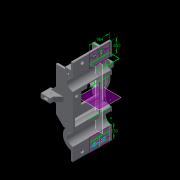
# Autodesk Inventor part: Extruder Holder V2
Saved by Autodesk Inventor 2014 (Build 180170000, 170)
## iProperties
Created: 2015-07-07
Part Number: Extruder Holder V2
Material: Generic
Document SubType Name: Modeling
Designer: Scott
Density: 1 g/cm^3
Appearance: Default
Author: Scott
Autodesk Inventor part; units mm, degrees
ref_plane "YZ Plane" through (0, 0, 0) normal (1, 0, 0) x (0, 1, 0)
ref_plane "XZ Plane" through (0, 0, 0) normal (0, 1, 0) x (-1, 0, 0)
ref_plane "XY Plane" through (0, 0, 0) normal (0, 0, 1) x (1, 0, 0)
ref_plane "Work Plane1" through (0, -60, 0) normal (0, 0, 1) x (-1, 0, 0)
sketch "Sketch1" plane through (0, -60, 0) normal (0, 0, 1) x (-1, 0, 0)
  circle A0 centre (0, 0) radius 4 projected
  circle A1 centre (0, -60) radius 4 projected
  circle A2 centre (0, -60) radius 7.5
  circle A3 centre (0, 0) radius 7.5
  circle A4 centre (0, -60) radius 12.7
  circle A5 centre (0, 0) radius 12.7
  dimension "d0" = 15
  dimension "d1" = 15
  dimension "d2" = 25.4
  dimension "d3" = 25.4
  constraints: 4 centre point, 4 coincident
  measures "d0" diameter of A2
  measures "d1" diameter of A3
  measures "d2" diameter of A4
  measures "d3" diameter of A5
extrude "Extrusion1" add sketch "Sketch1" along normal mid plane 25 contours A4 | A5
sketch "Sketch2" plane through (0, 0, 12.5) normal (0, 0, 1) x (1, 0, 0)
  circle A0 centre (0, 0) radius 12.7 projected
  circle A1 centre (0, -60) radius 7.5 projected
  circle A2 centre (0, -60) radius 12.7 projected
  circle A3 centre (0, 0) radius 7.5 projected
  circle A4 centre (0, 0) radius 12.7 projected
  line L0 (0, -72.7) -> (12.7, -72.7)
  line L1 (12.7, -72.7) -> (12.7, 12.706)
  line L2 (12.7, 12.706) -> (0, 12.7)
  circle A5 centre (0, -60) radius 12.7 projected
  arc A6 (0, -72.7) -> (12.7, -60) centre (0, -60) ccw
  arc A7 (12.7, 0) -> (0, 12.7) centre (0, 0) ccw
  constraints: 6 end point, 6 point on circle, 2 centre point, 2 horizontal, 2 point on line, 2 vertical alignment, 1 horizontal alignment, 1 perpendicular, 3 other
extrude "Extrusion2" add sketch "Sketch2" against normal blind 25 contours A0 L2 L1 | L1 L0 A2
sketch "Sketch3" plane through (12.7, 12.706, 12.5) normal (-0.0004741, 0.9999999, 0) x (0.9999999, 0.0004741, 0)
  line L0 (0, 0) -> (-12.7, 0) projected
  line L1 (0, 0) -> (0, 25) projected
  line L2 (-12.7, 25) -> (0, 25) projected
  line L3 (-12.7, 0) -> (-12.7, 25) projected
  point P0 (-12.706, 12.5)
sketch "Sketch4" plane through (0, -60, -12.5) normal (0, 0, -1) x (-1, 0, 0)
  line L0 (-12.7, 72.706) -> (-12.7, 60) projected
  line L1 (0, 72.7) -> (0, -16.7444)
  line L2 (0, -16.7444) -> (-14.0452, -16.7444)
  line L3 (-14.0452, -16.7444) -> (-14.0452, 76.9468)
  line L4 (-14.0452, 76.9468) -> (0, 72.7)
  constraints: 8 end point, 2 parallel, 1 perpendicular
extrude "Extrusion3" cut sketch "Sketch4" against normal blind 52.3875
sketch "Sketch5" plane through (0, 7.5, -12.5) normal (1, 0, 0) x (0, 0, -1)
  line L0 (-25, 0) -> (-25, 5.2) projected
  line L1 (0, 0) -> (-25, 0) projected
  line L2 (0, 5.2) -> (0, 0) projected
  line L3 (-25, 5.2) -> (0, 5.2) projected
  line L4 (-25, 0) -> (-0.0064, 0)
  line L5 (-0.0064, 0) -> (-0.0064, 16.51)
  line L6 (-0.0064, 16.51) -> (-25, 16.51)
  line L7 (-25, 16.51) -> (-25, 0)
  line L8 (-12.5, 5.2) -> (-12.5032, 16.51)
  line L9 (-12.5016, 10.855) -> (-25, 10.855)
  circle A0 centre (-18.7508, 10.855) radius 2.2225
  line L10 (-0.0064, 10.855) -> (-12.5016, 10.855)
  circle A1 centre (-6.254, 10.855) radius 2.2225
  line L11 (0, -20.2) -> (-25, -20.2) projected
  line L12 (-25, -54.8) -> (0, -54.8) projected
  line L13 (-12.5, -20.2) -> (-12.5, -54.8)
  line L14 (-12.5, -37.5) -> (-25, -37.5)
  line L15 (-25, -75) -> (0, -75) projected
  line L16 (-25, -80.2) -> (-25, -75) projected
  line L17 (-25, -80.2) -> (0, -80.2) projected
  line L18 (0, -75) -> (0, -80.2) projected
  line L19 (-25, -75) -> (0, -75)
  line L20 (0, -75) -> (0, -91.51)
  line L21 (0, -91.51) -> (-25, -91.51)
  line L22 (-25, -91.51) -> (-25, -75)
  line L23 (-12.5, -80.2) -> (-12.5, -91.51)
  line L24 (-25, -85.855) -> (-12.5, -85.855)
  line L25 (-12.5, -85.855) -> (0, -85.855)
  circle A2 centre (-18.75, -85.855) radius 2.2225
  circle A3 centre (-6.25, -85.855) radius 2.2225
  point P0 (-12.5, -7.5)
  dimension "d10" = 24.9936
  dimension "d11" = 16.51
  dimension "d12" = 4.445
  dimension "d13" = 4.445
  dimension "d14" = 16.51
  dimension "d15" = 4.445
  dimension "d16" = 4.445
  constraints: 32 end point, 13 midpoint, 5 perpendicular, 4 centre point, 4 parallel, 4 point on line, 2 horizontal, 1 collinear
  measures "d10" distance of L6.end L5.end
  measures "d11" distance of L5.end L4.end
  measures "d12" diameter of A0
  measures "d13" diameter of A1
  measures "d14" distance of L19.end L20.end
  measures "d15" diameter of A2
  measures "d16" diameter of A3
extrude "Extrusion4" add sketch "Sketch5" against normal blind 2.54
ref_plane "Work Plane2" through (0, -30, -12.5) normal (0, -1, 0) x (1, 0, 0)
sketch "Sketch6" plane through (0, -30, -12.5) normal (0, -1, 0) x (1, 0, 0)
  line L0 (0, 0) -> (0, 25) projected
  line L1 (0, 25) -> (0, 25) projected
  line L2 (0, 25) -> (0, 0) projected
  line L3 (0, 0) -> (0, 0) projected
  line L4 (-7.5, 25) -> (0, 25) projected
  line L5 (0, 0) -> (0, 25) projected
  line L6 (0, 25) -> (0, 25) projected
  line L7 (0, 25) -> (0, 0) projected
  line L8 (0, 0) -> (0, 0) projected
  line L9 (-2.54, 0) -> (-2.54, 25) projected
  line L10 (0, 25) -> (-2.54, 25) projected
  line L11 (0, 25) -> (0, 0) projected
  line L12 (-2.54, 0) -> (0, 0) projected
  line L13 (-7.5, 0) -> (-7.5, 25) projected
  line L14 (-7.5, 0) -> (-10.04, 0)
  line L15 (-10.04, 0) -> (-10.04, 43)
  line L16 (-7.5, 43) -> (-7.5, 0)
  line L17 (-10.04, 0) -> (-21.54, 0)
  line L18 (-21.54, 0) -> (-21.54, -2.54)
  line L19 (-21.54, -2.54) -> (-7.5, -2.54)
  line L20 (-7.5, -2.54) -> (-7.5, 0)
  line L21 (-10.04, 43) -> (-21.54, 43)
  line L22 (-21.54, 43) -> (-21.54, 45.54)
  line L23 (-21.54, 45.54) -> (-7.5, 45.54)
  line L24 (-7.5, 45.54) -> (-7.5, 43)
  point P0 (0, 12.5)
  dimension "d21" = 2.54
  dimension "d22" = 43
  dimension "d23" = 11.5
  dimension "d24" = 2.54
  dimension "d25" = 11.5
  dimension "d26" = 2.54
  constraints: 22 end point, 7 perpendicular, 3 parallel, 1 collinear
  measures "d21" distance of L13.start L14.end
  measures "d22" distance of L14.end L15.end
  measures "d23" distance of L14.end L17.end
  measures "d24" distance of L17.end L18.end
  measures "d25" distance of L15.end L21.end
  measures "d26" distance of L21.end L22.end
extrude "Extrusion6" add sketch "Sketch6" along normal blind 21.59 and the other way blind 42.2275 contours L14 L15 L21 L22 L23 L24 L16 L13 | L20 L19 L18 L17 L14
sketch "Sketch7" plane through (0, -51.59, -12.5) normal (0, -1, 0) x (1, 0, 0)
  line L0 (-10.04, 43) -> (-21.54, 43)
  line L1 (-21.54, 43) -> (-21.54, 0)
  line L2 (-21.54, 0) -> (-10.04, 0)
  line L3 (-10.04, 0) -> (-10.04, 43)
  point P0 (0, 12.5)
  constraints: 8 end point, 2 parallel, 1 horizontal, 1 perpendicular
extrude "Extrusion7" cut sketch "Sketch7" along normal mid plane 152.4
sketch "Sketch8" plane through (0, -60, 12.5) normal (0, 0, 1) x (1, 0, 0)
  line L0 (-7.5, 8.41) -> (-9.5164, 8.41) projected
  arc A0 (-9.5164, 8.41) -> (-2.54, -12.4434) centre (0, 0) ccw projected
  line L1 (-2.54, -24.01) -> (-2.54, -12.4434) projected
  line L2 (0, -24.01) -> (-2.54, -24.01) projected
  line L3 (0, -24.01) -> (0, -7.5) projected
  arc A1 (0, 7.5) -> (0, -7.5) centre (0, 0) ccw projected
  line L4 (0, 7.5) -> (0, 12.7) projected
  arc A2 (0, 12.7) -> (-7.5, 10.2489) centre (0, 0) ccw projected
  line L5 (-7.5, 10.2489) -> (-7.5, 8.41) projected
  line L6 (-7.5, 70.2489) -> (-7.5, 60) projected
  arc A3 (0, 67.5) -> (-7.5, 60) centre (0, 60) ccw projected
  line L7 (0, 84.01) -> (0, 67.5) projected
  line L8 (0, 84.01) -> (-2.54, 84.01) projected
  line L9 (-2.54, 72.4434) -> (-2.54, 84.01) projected
  arc A4 (-2.54, 72.4434) -> (-7.5, 70.2489) centre (0, 60) ccw projected
  line L10 (-7.5, 60) -> (-7.5, 49.7511) projected
  arc A5 (-7.5, 49.7511) -> (0, 47.3) centre (0, 60) ccw projected
  line L11 (0, 47.3) -> (0, 52.5) projected
  arc A6 (-7.5, 60) -> (0, 52.5) centre (0, 60) ccw projected
extrude "Extrusion8" add sketch "Sketch8" along normal up to surface (20.54 mm away)
sketch "Sketch9" plane through (0, -60, -12.5) normal (0, 0, -1) x (-1, 0, 0)
  line L0 (9.5164, 8.41) -> (7.5, 8.41) projected
  line L1 (7.5, 8.41) -> (7.5, 10.2489) projected
  arc A0 (7.5, 10.2489) -> (0, 12.7) centre (0, 0) ccw projected
  line L2 (0, 12.7) -> (0, 7.5) projected
  arc A1 (0, -7.5) -> (0, 7.5) centre (0, 0) ccw projected
  line L3 (0, -24.01) -> (0, -7.5) projected
  line L4 (0, -24.01) -> (2.54, -24.01) projected
  line L5 (2.54, -12.4434) -> (2.54, -24.01) projected
  arc A2 (2.54, -12.4434) -> (9.5164, 8.41) centre (0, 0) ccw projected
  arc A3 (8.3332, 63.0967) -> (2.2038, 68.6125) centre (0, 60) ccw projected
  line L6 (7.5, 60) -> (7.5, 70.2489) projected
  arc A4 (7.5, 70.2489) -> (2.54, 72.4434) centre (0, 60) ccw projected
  line L7 (2.54, 72.7) -> (2.54, 72.4434) projected
  line L8 (0, 72.7) -> (2.54, 72.7) projected
  line L9 (0, 72.7) -> (0, 67.5) projected
  arc A5 (7.5, 60) -> (0, 67.5) centre (0, 60) ccw projected
  line L10 (2.54, 72.7) -> (0, 72.7) projected
  line L11 (2.54, 84.01) -> (2.54, 72.7) projected
  line L12 (0, 84.01) -> (2.54, 84.01) projected
  line L13 (0, 72.7) -> (0, 84.01) projected
  line L14 (7.5, 49.7511) -> (7.5, 60) projected
  arc A6 (0, 52.5) -> (7.5, 60) centre (0, 60) ccw projected
  line L15 (0, 52.5) -> (0, 47.3) projected
  arc A7 (0, 47.3) -> (7.5, 49.7511) centre (0, 60) ccw projected
extrude "Extrusion9" add sketch "Sketch9" along normal up to surface (2.54 mm away)
sketch "Sketch10" plane through (-10.04, -51.59, -12.5) normal (-1, 0, 0) x (0, 0, 1)
  line L0 (43, 0) -> (33.221, 0)
  line L1 (33.221, 0) -> (33.221, 29.845)
  line L2 (33.221, 29.845) -> (43, 29.845)
  line L3 (43, 29.845) -> (43, 0)
  circle A0 centre (33.221, 29.845) radius 1.905
  line L4 (31.316, 29.845) -> (27.506, 29.845)
  line L5 (27.506, 29.845) -> (27.506, 42.545)
  line L6 (27.506, 42.545) -> (27.506, 17.145)
  line L7 (27.506, 17.145) -> (3.376, 17.145)
  line L8 (3.376, 17.145) -> (3.376, 42.545)
  line L9 (3.376, 42.545) -> (27.506, 42.545)
  point P0 (12.5, 51.59)
  dimension "d39" = 3.81
  dimension "d37" = 9.779
  dimension "d38" = 29.845
  dimension "d40" = 3.81
  dimension "d41" = 12.7
  dimension "d42" = 25.4
  dimension "d43" = 24.13
  constraints: 20 end point, 4 parallel, 4 perpendicular, 1 coincident, 1 collinear, 1 horizontal, 1 horizontal alignment, 2 other
  measures "d37" distance of L1.end L2.end
  measures "d38" distance of L0.end L1.end
  measures "d40" distance of L4.start L4.end
  measures "d41" distance of L4.end L5.end
  measures "d42" distance of L5.end L6.end
  measures "d43" distance of L6.end L7.end
extrude "Extrusion10" cut sketch "Sketch10" against normal blind 75.565 contours A0 L2 L1 | L1 L2 A0 | L6 L7 L8 L9 L5
sketch "Sketch11" plane through (-7.5, 12.2275, -15.04) normal (0, 0, -1) x (-1, 0, 0)
  arc A0 (-4.96, -84.6709) -> (2.0164, -63.8175) centre (-7.5, -72.2275) ccw projected
  line L0 (14.04, -63.8175) -> (2.0164, -63.8175) projected
  line L1 (-7.5, -24.9275) -> (-7.5, -21.2725) projected
  arc A1 (-7.5, -24.9275) -> (0, -22.4764) centre (-7.5, -12.2275) ccw projected
  line L2 (0, -46.6725) -> (0, -22.4764) projected
  line L3 (2.54, -46.6725) -> (0, -46.6725) projected
  line L4 (2.54, -21.2725) -> (2.54, -46.6725) projected
  line L5 (2.54, -21.2725) -> (-7.5, -21.2725) projected
  line L6 (2.54, 0) -> (2.54, -63.8175) projected
  line L7 (14.04, -63.8175) -> (2.54, -63.8175) projected
  line L8 (14.04, 0) -> (14.04, -63.8175) projected
  line L9 (2.54, 0) -> (14.04, 0) projected
  line L10 (2.54, -63.8175) -> (2.54, -64.4501)
  line L11 (2.54, -63.8175) -> (2.0164, -63.8175)
  line L12 (2.0164, -63.8175) -> (2.54, -64.4501)
  constraints: 6 end point, 1 collinear, 1 perpendicular, 1 point on circle
extrude "Extrusion11" add sketch "Sketch11" against normal up to surface (48.08 mm away) contours A0 L0 L10
fillet "Fillet1" radius 6.35 2 edges at (-7.5, -49.7511, -13.77) (-7.5, -49.7511, 10.27)
fillet "Fillet2" radius 6.35 2 edges at (-7.5, 10.2489, 10.27) (-7.5, 10.2489, -13.77)
chamfer "Chamfer1" distance 9.525 angle 45 2 edges at (-21.54, -51.59, -13.77) (-21.54, -51.59, 31.77)
sketch "Sketch14" plane through (0, -60, 33.04) normal (0, 0, 1) x (1, 0, 0)
  line L0 (-7.5, 49.7511) -> (-7.5, 19.0153) projected
  line L1 (-21.54, 72.2275) -> (-21.54, 17.935) projected
  line L2 (-10.04, 36.35) -> (-10.04, 40.16) projected
  line L3 (-10.04, 38.255) -> (-7.5, 38.255)
  line L4 (-7.5, 38.255) -> (-11.0275, 38.255)
  line L5 (-11.0275, 38.255) -> (-21.1875, 38.255)
  line L6 (-21.54, 38.255) -> (-27.382, 38.255)
  line L7 (-27.382, 36.985) -> (-21.54, 36.985)
  line L8 (-21.54, 36.985) -> (-21.54, 39.525)
  line L9 (-21.54, 39.525) -> (-27.382, 39.525)
  line L10 (-27.382, 39.525) -> (-27.382, 36.985)
  line L11 (-27.382, 36.985) -> (-21.54, 39.525) construction
  line L12 (-21.54, 36.985) -> (-27.382, 39.525) construction
  line L13 (-30.3665, 35.3975) -> (-18.5555, 35.3975)
  line L14 (-18.5555, 35.3975) -> (-18.5555, 41.1125)
  line L15 (-18.5555, 41.1125) -> (-30.3665, 41.1125)
  line L16 (-30.3665, 41.1125) -> (-30.3665, 35.3975)
  line L17 (-30.3665, 35.3975) -> (-18.5555, 41.1125) construction
  line L18 (-18.5555, 35.3975) -> (-30.3665, 41.1125) construction
  point P0 (-24.461, 38.255)
  dimension "d61" = 10.16
  dimension "d62" = 5.842
  dimension "d63" = 5.842
  dimension "d64" = 2.54
  dimension "d65" = 11.811
  dimension "d66" = 5.715
  constraints: 32 end point, 6 midpoint, 4 parallel, 3 collinear, 3 perpendicular, 2 horizontal, 2 point on line
  measures "d61" distance of L4.end L5.end
  measures "d62" distance of L6.start L6.end
  measures "d63" distance of L9.end L8.end
  measures "d64" distance of L8.end L7.end
  measures "d65" distance of L15.end L14.end
  measures "d66" distance of L14.end L13.end
extrude "Extrusion14" add sketch "Sketch14" along normal blind 10.16 contours L1 L15 L14 L13 | L9 L10 L7 L1 L13 L16 L15
sketch "Sketch15" plane through (0, -60, 33.04) normal (0, 0, -1) x (-1, 0, 0)
  line L0 (30.3665, 41.1125) -> (21.54, 41.1125)
  line L1 (21.54, 41.1125) -> (21.54, 35.3975)
  line L2 (21.54, 35.3975) -> (30.3665, 35.3975)
  line L3 (30.3665, 35.3975) -> (30.3665, 41.1125)
  point P0 (0, 60)
  constraints: 8 end point, 2 parallel, 1 horizontal, 1 perpendicular
extrude "Extrusion15" add sketch "Sketch15" along normal up to surface (2.54 mm away)
chamfer "Chamfer2" distance 6.35 angle 45 1 edges at (-18.5555, -21.745, 33.04)
chamfer "Chamfer3" distance 6.35 angle 45 2 edges at (-21.54, -24.6025, 31.77) (-21.54, -18.8875, 31.77)
sketch "Sketch16" plane through (0, 0, -15.04) normal (0, 0, -1) x (-1, 0, 0)
  line L0 (21.54, -42.065) -> (12.015, -51.59) projected
  line L1 (21.54, 12.2275) -> (21.54, -42.065) projected
  line L2 (7.5, 12.2275) -> (21.54, 12.2275) projected
  arc A0 (3.6503, 12.1641) -> (7.5, 12.2275) centre (5.4755, 18.2461) ccw projected
  arc A1 (3.6503, 12.1641) -> (2.54, 12.4434) centre (0, 0) ccw projected
  line L3 (2.54, 24.01) -> (2.54, 12.4434) projected
  line L4 (0, 24.01) -> (2.54, 24.01) projected
  line L5 (0, 7.5) -> (0, 24.01) projected
  arc A2 (0, -7.5) -> (0, 7.5) centre (0, 0) ccw projected
  line L6 (0, -12.7) -> (0, -7.5) projected
  arc A3 (0, -12.7) -> (7.5, -10.2489) centre (0, 0) ccw projected
  line L7 (7.5, -10.2489) -> (7.5, -40.9847) projected
  arc A4 (0.7667, -47.3232) -> (7.5, -40.9847) centre (1.15, -40.9847) ccw projected
  arc A5 (0.7667, -47.3232) -> (0, -47.3) centre (0, -60) ccw projected
  line L8 (0, -52.5) -> (0, -47.3) projected
  arc A6 (0, -67.5) -> (0, -52.5) centre (0, -60) ccw projected
  line L9 (0, -84.01) -> (0, -67.5) projected
  line L10 (2.54, -84.01) -> (0, -84.01) projected
  line L11 (2.54, -72.4434) -> (2.54, -84.01) projected
  arc A7 (2.54, -72.4434) -> (10.04, -52.2226) centre (0, -60) ccw projected
  line L12 (10.04, -52.2226) -> (10.04, -51.59) projected
  line L13 (12.015, -51.59) -> (10.04, -51.59) projected
  line L14 (11, -18.441) -> (11, -2.5) projected
sketch "Sketch17" plane through (-21.54, 12.2275, -15.04) normal (-1, 0, 0) x (0, 0, 1)
  line L0 (2.54, 0) -> (2.54, -54.2925) projected
  line L1 (0, 0) -> (0, -54.2925) projected
  line L2 (5.916, -21.2725) -> (30.046, -21.2725) projected
  line L3 (30.046, -46.6725) -> (5.916, -46.6725) projected
  line L4 (0, -21.2725) -> (-7.62, -21.2725)
  line L5 (-7.62, -21.2725) -> (-7.62, -46.6725)
  line L6 (-7.62, -46.6725) -> (0, -46.6725)
  line L7 (0, -46.6725) -> (0, -21.2725)
  line L8 (0, -21.2725) -> (0, -17.4625)
  line L9 (0, -17.4625) -> (-11.43, -17.4625)
  line L10 (-11.43, -17.4625) -> (-11.43, -46.6725)
  line L11 (-11.43, -46.6725) -> (-11.43, -50.4825)
  line L12 (-11.43, -50.4825) -> (0, -50.4825)
  line L13 (0, -21.8952) -> (2.54, -21.8952)
  line L14 (0, -17.4625) -> (2.54, -17.4625)
  line L15 (2.54, -21.8952) -> (2.54, -17.4625)
  line L16 (0, -50.4825) -> (2.54, -50.4825)
  line L17 (0, -46.6725) -> (2.54, -46.6725)
  line L18 (2.54, -46.6725) -> (2.54, -50.4825)
  line L19 (0, -21.2725) -> (2.54, -21.2725)
  point P0 (15.04, -12.2275)
  dimension "d77" = 7.62
  dimension "d78" = 25.4
  dimension "d79" = 3.81
  dimension "d80" = 11.43
  dimension "d81" = 3.81
  constraints: 32 end point, 9 point on line, 8 perpendicular, 4 parallel, 2 collinear, 1 horizontal
  measures "d77" distance of L6.end L5.end
  measures "d78" distance of L5.end L4.end
  measures "d79" distance of L4.start L8.end
  measures "d80" distance of L8.end L9.end
  measures "d81" distance of L10.end L11.end
extrude "Extrusion16" add sketch "Sketch17" along normal mid plane 18.0975 contours L0 L19 L1 L14 | L1 L4 L5 L6 L12 L11 L10 L9 | L0 L16 L1 L17
sketch "Sketch18" plane through (-30.5888, -9.045, -22.66) normal (0, 0, 1) x (1, 0, 0)
  line L0 (3.2068, -13.97) -> (3.2068, -11.43) projected
  line L1 (3.2068, -11.43) -> (9.0488, -11.43) projected
  line L2 (9.0488, -11.43) -> (9.0488, -13.97) projected
  line L3 (9.0488, -13.97) -> (3.2068, -13.97) projected
  line L4 (0.2223, -15.5575) -> (12.0332, -15.5575) projected
  line L5 (12.0332, -15.5575) -> (12.0332, -9.8425) projected
  line L6 (12.0332, -9.8425) -> (0.2223, -9.8425) projected
  line L7 (0.2223, -9.8425) -> (0.2223, -15.5575) projected
  point P0 (30.5888, 9.045)
extrude "Extrusion17" add sketch "Sketch18" against normal blind 13.97
sketch "Sketch19" plane through (-21.54, -34.445, -12.5) normal (-1, 0, 0) x (0, 0, 1)
  line L0 (-2.54, 0) -> (0, 0) projected
  line L1 (0, 25.4) -> (0, 0) projected
  line L2 (0, 25.4) -> (-2.54, 25.4) projected
  line L3 (-2.54, 25.4) -> (-2.54, 0) projected
  line L4 (-2.54, 21.745) -> (3.376, 21.745) projected
  line L5 (-2.54, 0) -> (0, 0) projected
  line L6 (0, 25.4) -> (0, 0) projected
  line L7 (0, 25.4) -> (-2.54, 25.4) projected
  line L8 (-2.54, 25.4) -> (-2.54, 0) projected
  point P0 (12.5, 34.445)
extrude "Extrusion18" cut sketch "Sketch19" against normal blind 6.0325
fillet "Fillet3" radius 7.9375 8 edges at (-17.0156, -34.445, -22.66) (-26.0644, -34.445, -22.66) (-17.0156, -38.255, -26.47) (-26.0644, -38.255, -26.47) (-17.0156, -5.235, -26.47) (-26.0644, -5.235, -26.47) (-17.0156, -9.045, -22.66) (-26.0644, -9.045, -22.66)
chamfer "Chamfer5" distance 4.7625 angle 45 2 edges at (-12.4912, -7.1432, -15.04) (-12.4912, -36.3468, -15.04)
chamfer "Chamfer6" distance 7.9375 angle 45 1 edges at (-21.54, -5.235, -13.77)
chamfer "Chamfer7" distance 4.7625 angle 45 1 edges at (-18.5555, -21.745, -26.47)
chamfer "Chamfer8" distance 6.35 angle 45 2 edges at (-30.5888, -36.35, -12.5) (-30.5888, -7.14, -12.5)
sketch "Sketch20" plane through (0, -60, 33.04) normal (0, 0, 1) x (1, 0, 0)
  arc A0 (-7.5, 19.0153) -> (-0.7667, 12.6768) centre (-1.15, 19.0153) ccw projected
  line L0 (-5.0623, 14.0136) -> (-8.4175, 14.0136)
  line L1 (-8.4175, 14.0136) -> (-8.4175, 19.653)
  line L2 (-8.4175, 19.653) -> (-5.0623, 19.653)
  line L3 (-5.0623, 19.653) -> (-5.0623, 14.0136)
  constraints: 8 end point, 2 parallel, 1 horizontal, 1 perpendicular, 1 point on circle
extrude "Extrusion19" cut sketch "Sketch20" against normal blind 56.8325
sketch "Sketch21" plane through (-10.04, 12.2275, 30.5) normal (0, 0, -1) x (-1, 0, 0)
  line L0 (21.1166, -48.5775) -> (21.1166, -35.8775) projected
  line L1 (0.96, -35.8775) -> (21.1166, -35.8775) projected
  line L2 (0.96, -48.5775) -> (21.1166, -48.5775) projected
  line L3 (21.1166, -48.5775) -> (11.5, -48.5775)
  line L4 (11.5, -48.5775) -> (11.5, -54.2925)
  line L5 (11.5, -54.2925) -> (21.1166, -54.2925)
  line L6 (21.1166, -54.2925) -> (21.1166, -48.5775)
  point P0 (-10.04, -12.2275)
  constraints: 8 end point, 2 parallel, 1 horizontal, 1 perpendicular
extrude "Extrusion20" cut sketch "Sketch21" along normal blind 56.8325
fillet "Fillet4" radius 1.5875 1 edges at (-21.54, -36.35, -18.0956)
sketch "Sketch22" plane through (-30.3665, -24.6025, -36.63) normal (0, -1, 0) x (1, 0, 0)
  circle A0 centre (5.9055, 5.08) radius 0.635
  line L0 (2.4765, 69.67) -> (2.4765, 67.13) projected
  line L1 (2.4765, 69.67) -> (18.161, 69.67) projected
  line L2 (11.811, 76.02) -> (18.161, 69.67) projected
  line L3 (11.811, 76.02) -> (11.811, 79.83) projected
  line L4 (0, 79.83) -> (11.811, 79.83) projected
  line L5 (0, 79.83) -> (0, 67.13) projected
  line L6 (0, 67.13) -> (2.4765, 67.13) projected
  circle A1 centre (6.5405, 73.48) radius 0.635
  point P0 (30.3665, 36.63)
  dimension "d109" = 1.27
  dimension "d110" = 1.27
  constraints: 2 centre point
  measures "d109" diameter of A0
  measures "d110" diameter of A1
extrude "Extrusion21" cut sketch "Sketch22" against normal blind 56.8325 contours A0 | A1
sketch "Sketch23" plane through (-2.54, 7.5, -12.5) normal (-1, 0, 0) x (0, 0, 1)
  line L0 (-2.54, -79.9434) -> (45.54, -79.9434) projected
  line L1 (-2.54, -79.9434) -> (-2.54, -91.51) projected
  line L2 (45.54, -91.51) -> (-2.54, -91.51) projected
  line L3 (45.54, -91.51) -> (45.54, -79.9434) projected
  line L4 (45.54, 4.9434) -> (-2.54, 4.9434) projected
  line L5 (45.54, 4.9434) -> (45.54, 16.51) projected
  line L6 (0.0064, 16.51) -> (45.54, 16.51) projected
  line L7 (0.0064, 16.51) -> (0.0064, 5.2) projected
  line L8 (0.0064, 5.2) -> (0, 5.2) projected
  line L9 (0, 5.2) -> (0, 16.51) projected
  line L10 (0, 16.51) -> (-2.54, 16.51) projected
  line L11 (-2.54, 16.51) -> (-2.54, 4.9434) projected
  line L12 (21.5, -79.9434) -> (21.5, -91.51)
  line L13 (21.5, -85.7267) -> (45.54, -85.7267)
  line L14 (21.5, -85.7267) -> (-2.54, -85.7267)
  circle A0 centre (9.48, -85.7267) radius 2.2225
  circle A1 centre (33.52, -85.7267) radius 2.2225
  line L15 (21.5, 16.51) -> (21.5, 4.9434)
  line L16 (21.5, 10.7267) -> (-2.54, 10.7267)
  line L17 (21.5, 10.7267) -> (45.54, 10.7267)
  circle A2 centre (9.48, 10.7267) radius 2.2225
  circle A3 centre (33.52, 10.7267) radius 2.2225
  point P0 (12.5, -7.5)
  dimension "d113" = 4.445
  dimension "d114" = 4.445
  dimension "d115" = 4.445
  dimension "d116" = 4.445
  constraints: 13 midpoint, 12 end point, 4 centre point, 1 point on line
  measures "d113" diameter of A0
  measures "d114" diameter of A1
  measures "d115" diameter of A2
  measures "d116" diameter of A3
extrude "Extrusion22" cut sketch "Sketch23" against normal blind 56.8325 contours A0 L14 | L14 A0 | A1 L13 | L13 A1 | A3 L17 | L17 A3 | A2 L16 | L16 A2
chamfer "Chamfer9" distance 1.5875 angle 45 3 edges at (-12.4912, -21.745, -22.66) (-12.4912, -29.8751, -21.9102) (-12.4912, -13.6149, -21.9102)
chamfer "Chamfer10" distance 3.175 angle 45 2 edges at (-14.6344, -38.255, -15.04) (-17.2537, -5.235, -15.04)
sketch "Sketch24" plane through (-7.5, -34.445, -9.124) normal (1, 0, 0) x (0, 0, -1)
  line L0 (-24.13, 24.1961) -> (-42.164, 24.1961) projected
  line L1 (5.916, -18.055) -> (-42.164, -18.055) projected
  line L2 (5.916, -18.055) -> (5.916, -12.855) projected
  line L3 (-42.164, -12.855) -> (5.916, -12.855) projected
  line L4 (-42.164, -12.855) -> (-42.164, -18.055) projected
  line L5 (-42.164, -12.855) -> (-39.624, -12.855)
  line L6 (-39.624, -12.855) -> (-39.624, 24.1961)
  line L7 (-39.624, 24.1961) -> (-42.164, 24.1961)
  line L8 (-42.164, 24.1961) -> (-42.164, -12.855)
  point P0 (-9.124, 34.445)
  dimension "d125" = 2.54
  constraints: 8 end point, 2 parallel, 1 horizontal, 1 perpendicular, 1 point on line
  measures "d125" distance of L7.end L6.end
extrude "Extrusion23" add sketch "Sketch24" along normal up to surface (7.5 mm away) contours L6 L3 L8 L0
sketch "Sketch25" plane through (0, 0, -15.04) normal (0, 0, -1) x (-1, 0, 0)
  line L0 (7.5, 12.2275) -> (4.96, 12.2275)
  line L1 (4.96, 12.2275) -> (4.96, 8.4175)
  line L2 (4.96, 8.4175) -> (7.5, 8.4175)
  line L3 (7.5, 8.4175) -> (7.5, 12.2275)
  dimension "d128" = 2.54
  dimension "d129" = 3.81
  constraints: 8 end point, 2 parallel, 1 horizontal, 1 perpendicular
  measures "d128" distance of L2.end L1.end
  measures "d129" distance of L1.end L0.end
sketch "Sketch26" plane through (0, -60, 0) normal (0, 0, 1) x (-1, 0, 0)
  line L0 (7.5, -68.4175) -> (7.5, -72.2275) projected
  line L1 (4.96, -68.4175) -> (7.5, -68.4175) projected
  line L2 (7.5, -72.2275) -> (4.96, -72.2275) projected
  line L3 (4.96, -72.2275) -> (4.96, -68.4175) projected
  line L4 (7.5, -68.4175) -> (10.04, -68.4175)
  line L5 (10.04, -68.4175) -> (10.04, -72.2275)
  line L6 (10.04, -72.2275) -> (10.04, -74.7675)
  line L7 (10.04, -74.7675) -> (2.5022, -74.7675)
  line L8 (2.5022, -74.7675) -> (2.5022, -68.4175)
  line L9 (2.5022, -68.4175) -> (10.04, -68.4175)
  point P0 (0, -60)
  dimension "d130" = 2.54
  dimension "d131" = 2.54
  constraints: 12 end point, 2 collinear, 2 parallel, 2 perpendicular
  measures "d130" distance of L0.start L4.end
  measures "d131" distance of L5.end L6.end
extrude "Extrusion24" add sketch "Sketch26" against normal up to surface (48.08 mm away) from surface at 33.04 contours L4 L5 L6 L7 L8 L9 L3 L2 L0
extrude "Extrusion25" cut sketch "Sketch25" against normal blind 56.8325
sketch "Sketch27" plane through (-2.54, 7.5, -12.5) normal (-1, 0, 0) x (0, 0, 1)
  circle A0 centre (9.48, 10.7267) radius 2.2225 projected
  circle A1 centre (33.52, 10.7267) radius 2.2225 projected
  circle A2 centre (9.48, 10.7267) radius 4.445
  circle A3 centre (33.52, 10.7267) radius 4.445
  point P0 (12.5, -7.5)
  dimension "d136" = 8.89
  dimension "d137" = 8.89
  constraints: 2 centre point, 2 coincident
  measures "d136" diameter of A2
  measures "d137" diameter of A3
extrude "Extrusion26" cut sketch "Sketch27" along normal blind 56.8325
body "Solid1"
